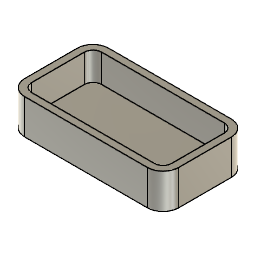
Box project (Autodesk Fusion 360 design; units mm, degrees)
part number: 2025-07-20-15-59-06-694
part number: 2025-07-20-16-55-08-906
part number: 2025-07-20-16-55-23-234
part number: 2025-07-20-16-56-02-410
Autodesk Fusion 360 part; units mm, degrees
note: some values were not read from the file. Chosen so that the rebuilt part matches the saved one: which face or edge a step refers to.
sketch "Sketch1" plane through (0, 0, 0) normal (0, 0, 1) x (1, 0, 0) in component "Box"
  line L0 (88.9, -50.8) -> (-88.9, -50.8)
  line L1 (-101.6, -38.1) -> (-101.6, 38.1)
  line L2 (-88.9, 50.8) -> (88.9, 50.8)
  line L3 (101.6, 38.1) -> (101.6, -38.1)
  line L4 (101.6, -50.8) -> (-101.6, 50.8) construction
  line L5 (-101.6, -50.8) -> (101.6, 50.8) construction
  arc A0 (-88.9, 50.8) -> (-101.6, 38.1) centre (-88.9, 38.1) ccw
  arc A1 (101.6, 38.1) -> (88.9, 50.8) centre (88.9, 38.1) ccw
  arc A2 (88.9, -50.8) -> (101.6, -38.1) centre (88.9, -38.1) ccw
  arc A3 (-101.6, -38.1) -> (-88.9, -50.8) centre (-88.9, -38.1) ccw
  arc A4 (111.76, 38.1) -> (88.9, 60.96) centre (88.9, 38.1) ccw
  line L6 (-88.9, 60.96) -> (88.9, 60.96)
  arc A5 (-88.9, 60.96) -> (-111.76, 38.1) centre (-88.9, 38.1) ccw
  line L7 (-111.76, -38.1) -> (-111.76, 38.1)
  arc A6 (-111.76, -38.1) -> (-88.9, -60.96) centre (-88.9, -38.1) ccw
  line L8 (88.9, -60.96) -> (-88.9, -60.96)
  arc A7 (88.9, -60.96) -> (111.76, -38.1) centre (88.9, -38.1) ccw
  line L9 (111.76, 38.1) -> (111.76, -38.1)
  dimension "d1" = 203.2
  dimension "d2" = 101.6
  dimension "d3" = 12.7
  dimension "d4" = -10.16
  constraint horizontal L0
  constraint perpendicular L0 L1
  constraint parallel L0 L2
  constraint parallel L1 L3
  constraint coincident L4 origin
  constraint coincident L5 origin
  constraint coincident L4.end L1
  constraint coincident L4.end L2
  constraint tangent L1 A0
  constraint tangent L2 A0
  constraint coincident L5.end L2
  constraint coincident L5.end L3
  constraint tangent L2 A1
  constraint tangent L3 A1
  constraint equal A0 A1
  constraint coincident L4.start L3
  constraint coincident L4.start L0
  constraint tangent L3 A2
  constraint tangent L0 A2
  constraint equal A0 A2
  constraint coincident L5.start L0
  constraint coincident L5.start L1
  constraint tangent L0 A3
  constraint tangent L1 A3
  constraint equal A0 A3
  measures "d1" distance of L4.end L5.end
  measures "d2" distance of L5.start L4.end
  measures "d3" radius of A0
extrude "Extrude1" add sketch "Sketch1" along normal blind 50.8 makes body 1 in component "Screew"
copy_body "CutPasteBodies1" bodies 1 removing the originals makes body 2 in component "Box"
extrude "Extrude1'" add sketch "Sketch1" along normal blind 10.16 contours L0 L1 L2 L3 A0 A1 A2 A3 bodies 2 in component "Box"
sketch "Sketch1 (1)" plane through (0, 0, 10.16) normal (0, 0, 1) x (-1, 0, 0) in component "Box"
  arc A0 (88.9, -50.8) -> (101.6, -38.1) centre (88.9, -38.1) ccw
  line L0 (101.6, -38.1) -> (101.6, 38.1)
  arc A1 (101.6, 38.1) -> (88.9, 50.8) centre (88.9, 38.1) ccw
  line L1 (88.9, 50.8) -> (-88.9, 50.8)
  arc A2 (-88.9, 50.8) -> (-101.6, 38.1) centre (-88.9, 38.1) ccw
  line L2 (-101.6, 38.1) -> (-101.6, -38.1)
  arc A3 (-101.6, -38.1) -> (-88.9, -50.8) centre (-88.9, -38.1) ccw
  line L3 (-88.9, -50.8) -> (88.9, -50.8)
  line L4 (100.33, 52.07) -> (-100.33, 52.07)
  line L5 (-100.33, 52.07) -> (-100.33, -52.07)
  line L6 (-100.33, -52.07) -> (100.33, -52.07)
  line L7 (100.33, -52.07) -> (100.33, 52.07)
  line L8 (100.33, 52.07) -> (-100.33, -52.07) construction
  line L9 (-100.33, 52.07) -> (100.33, -52.07) construction
  dimension "d9" = 200.66
  dimension "d10" = 104.14
  constraint horizontal L4
  constraint perpendicular L4 L5
  constraint parallel L4 L6
  constraint parallel L5 L7
  constraint coincident L8 origin
  constraint coincident L9 origin
  measures "d9" distance of L5.end L6.end
  measures "d10" distance of L4.end L5.end
hole "Hole1" at (100.33, 52.07, 10.16) at (100.33, -52.07, 10.16) at (-100.33, -52.07, 10.16) at (-100.33, 52.07, 10.16) direction (0, 0, -1) diameter 6.57 depth 25.4 tip angle 118 bodies 2 in component "Box"
thread "Thread1" "ANSI Unified Screw Threads 0.3125 5/16-18 UNC 5/16-18 UNC 1B" major diameter 7.9375 minor diameter 6.5659 pitch 1.4111 angle 60 resizes the face on face at (-102.0429, -54.8731, 6.7733) on face at (98.6171, -54.8731, 6.7733) on face at (-102.0429, 49.2669, 6.7733) on face at (98.6171, 49.2669, 6.7733) on bodies 2 in component "Box"
component "Lid" placed x (1, 0, 0) y (0, 1, 0) z (0, 0, 1) at (0, 0, 0)
component "Box" placed x (1, 0, 0) y (0, 1, 0) z (0, 0, 1) at (0, 0, 0)
component "Screew" placed x (1, 0, 0) y (0, 1, 0) z (0, 0, 1) at (0, 0, 0)
